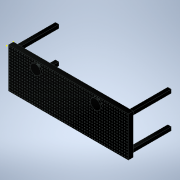
# Autodesk Inventor part: Table_Holed
Saved by Autodesk Inventor 2020 (Build 240168000, 168)
## iProperties
Created: 2019-11-01
Part Number: Table_Holed
Material: Generic
Document SubType Name: Modeling
Designer: Nikol
Density: 1 g/cm^3
Appearance: Gunmetal - Polished
Author: Nikol
Autodesk Inventor part; units mm, degrees
ref_plane "YZ Plane" through (0, 0, 0) normal (1, 0, 0) x (0, 1, 0)
ref_plane "XZ Plane" through (0, 0, 0) normal (0, 1, 0) x (-1, 0, 0)
ref_plane "XY Plane" through (0, 0, 0) normal (0, 0, 1) x (1, 0, 0)
sketch "Sketch1" plane through (0, 0, 0) normal (0, 0, 1) x (1, 0, 0)
  line L0 (0, 0) -> (2400, 0)
  line L1 (2400, 0) -> (2400, -800)
  line L2 (2400, -800) -> (0, -800)
  line L3 (0, -800) -> (0, 0)
  line L4 (0, 0) -> (575, 0)
  line L5 (575, 0) -> (575, -125)
  line L6 (0, 0) -> (1775, 0)
  line L7 (1775, 0) -> (1775, -125)
  circle A0 centre (575, -125) radius 100
  circle A1 centre (1775, -125) radius 100
  dimension "d0" = 2400
  dimension "d1" = 800
  dimension "d2" = 575
  dimension "d3" = 125
  dimension "d4" = 1775
  dimension "d5" = 200
  constraints: 16 end point, 3 perpendicular, 2 centre point, 2 coincident, 2 parallel, 2 point on line, 1 horizontal
  measures "d0" distance of L1.end L2.end
  measures "d1" distance of L0.end L1.end
  measures "d2" distance of L0.start L4.end
  measures "d3" distance of L4.end L5.end
  measures "d4" distance of L0.start L6.end
  measures "d5" diameter of A0
extrude "Extrusion1" add sketch "Sketch1" along normal blind 35 contours A1 | A0
extrude "Extrusion2" add sketch "Sketch1" against normal blind 100
sketch "Sketch2" plane through (575, -125, 35) normal (0, 0, 1) x (1, 0, 0)
  point P0 (-575, 125)
extrude "Extrusion3" add sketch "Sketch1" against normal blind 100 contours A0
extrude "Extrusion4" add sketch "Sketch1" against normal blind 100 contours A1
sketch "Sketch3" plane through (0, 0, -100) normal (0, 0, -1) x (-1, 0, 0)
  point P0 (0, 0)
sketch "Sketch4" plane through (0, 0, -100) normal (0, 0, -1) x (-1, 0, 0)
  line L0 (0, 0) -> (-2400, 0) projected
  line L1 (0, 0) -> (0, -40)
  line L2 (0, -800) -> (0, 0) projected
  line L3 (0, -40) -> (-40, -40)
  line L4 (-40, -40) -> (-110, -40)
  line L5 (-110, -40) -> (-110, -110)
  line L6 (-110, -110) -> (-40, -110)
  line L7 (-40, -110) -> (-40, -40)
  line L8 (-2400, -800) -> (0, -800) projected
  line L9 (0, -800) -> (-40, -800)
  line L10 (0, -760) -> (0, -800)
  line L11 (-40, -760) -> (-110, -760)
  line L12 (-110, -760) -> (-110, -690)
  line L13 (-110, -690) -> (-40, -690)
  line L14 (-40, -690) -> (-40, -760)
  line L15 (-2400, 0) -> (-2400, -800) projected
  line L16 (-2400, 0) -> (-2400, -40)
  line L17 (-2400, -40) -> (-2360, -40)
  line L18 (-2400, -800) -> (-2400, -760)
  line L19 (-2400, -760) -> (-2360, -760)
  line L20 (-2360, -40) -> (-2290, -40)
  line L21 (-2290, -40) -> (-2290, -110)
  line L22 (-2290, -110) -> (-2360, -110)
  line L23 (-2360, -110) -> (-2360, -40)
  line L24 (-2360, -760) -> (-2290, -760)
  line L25 (-2290, -760) -> (-2290, -690)
  line L26 (-2290, -690) -> (-2360, -690)
  line L27 (-2360, -690) -> (-2360, -760)
  dimension "d14" = 40
  dimension "d15" = 40
  dimension "d16" = 70
  dimension "d17" = 70
  dimension "d18" = 40
  dimension "d19" = 40
  dimension "d20" = 70
  dimension "d21" = 70
  dimension "d22" = 40
  dimension "d23" = 40
  dimension "d24" = 70
  dimension "d25" = 70
  dimension "d26" = 70
  dimension "d27" = 70
  constraints: 48 end point, 8 parallel, 6 horizontal, 6 perpendicular, 3 point on line
  measures "d14" distance of L0.start L1.end
  measures "d15" distance of L1.end L3.end
  measures "d16" distance of L6.end L5.end
  measures "d17" distance of L5.end L4.end
  measures "d18" distance of L11.start L10.start
  measures "d19" distance of L9.end L11.start
  measures "d20" distance of L12.end L13.end
  measures "d21" distance of L11.end L12.end
  measures "d22" distance of L0.end L16.end
  measures "d23" distance of L16.end L17.end
  measures "d24" distance of L21.end L22.end
  measures "d25" distance of L20.end L21.end
  measures "d26" distance of L26.end L25.end
  measures "d27" distance of L25.end L24.end
extrude "Extrusion5" add sketch "Sketch4" along normal blind 800 contours L20 L21 L22 L23 | L27 L26 L25 L24 | L7 L6 L5 L4 | L11 L12 L13 L14
sketch "Sketch5" plane through (0, 0, 0) normal (0, 0, 1) x (1, 0, 0)
  circle A0 centre (25, -25) radius 10
  circle A1 centre (25, -75) radius 10
  circle A2 centre (25, -175) radius 10
  circle A3 centre (25, -125) radius 10
  circle A4 centre (25, -375) radius 10
  circle A5 centre (25, -325) radius 10
  circle A6 centre (25, -225) radius 10
  circle A7 centre (25, -275) radius 10
  circle A8 centre (25, -775) radius 10
  circle A9 centre (25, -725) radius 10
  circle A10 centre (25, -625) radius 10
  circle A11 centre (25, -675) radius 10
  circle A12 centre (25, -425) radius 10
  circle A13 centre (25, -475) radius 10
  circle A14 centre (25, -575) radius 10
  circle A15 centre (25, -525) radius 10
  line L0 (2400, -800) -> (0, -800) projected
  circle A16 centre (75, -25) radius 10
  circle A17 centre (75, -75) radius 10
  circle A18 centre (75, -175) radius 10
  circle A19 centre (75, -125) radius 10
  circle A20 centre (75, -375) radius 10
  circle A21 centre (75, -325) radius 10
  circle A22 centre (75, -225) radius 10
  circle A23 centre (75, -275) radius 10
  circle A24 centre (75, -525) radius 10
  circle A25 centre (75, -475) radius 10
  circle A26 centre (75, -425) radius 10
  circle A27 centre (75, -775) radius 10
  circle A28 centre (75, -575) radius 10
  circle A29 centre (75, -625) radius 10
  circle A30 centre (75, -675) radius 10
  circle A31 centre (75, -725) radius 10
  circle A32 centre (125, -625) radius 10
  circle A33 centre (125, -725) radius 10
  circle A34 centre (125, -575) radius 10
  circle A35 centre (125, -525) radius 10
  circle A36 centre (125, -475) radius 10
  circle A37 centre (125, -425) radius 10
  circle A38 centre (125, -375) radius 10
  circle A39 centre (125, -325) radius 10
  circle A40 centre (125, -275) radius 10
  circle A41 centre (125, -225) radius 10
  circle A42 centre (125, -125) radius 10
  circle A43 centre (125, -75) radius 10
  circle A44 centre (125, -25) radius 10
  circle A45 centre (125, -175) radius 10
  circle A46 centre (125, -675) radius 10
  circle A47 centre (125, -775) radius 10
  circle A48 centre (275, -25) radius 10
  circle A49 centre (275, -75) radius 10
  circle A50 centre (275, -175) radius 10
  circle A51 centre (275, -125) radius 10
  circle A52 centre (275, -375) radius 10
  circle A53 centre (275, -325) radius 10
  circle A54 centre (275, -225) radius 10
  circle A55 centre (275, -275) radius 10
  circle A56 centre (275, -525) radius 10
  circle A57 centre (275, -475) radius 10
  circle A58 centre (275, -425) radius 10
  circle A59 centre (275, -775) radius 10
  circle A60 centre (275, -575) radius 10
  circle A61 centre (275, -625) radius 10
  circle A62 centre (275, -675) radius 10
  circle A63 centre (275, -725) radius 10
  circle A64 centre (225, -625) radius 10
  circle A65 centre (225, -725) radius 10
  circle A66 centre (225, -575) radius 10
  circle A67 centre (225, -525) radius 10
  circle A68 centre (225, -475) radius 10
  circle A69 centre (225, -425) radius 10
  circle A70 centre (225, -375) radius 10
  circle A71 centre (225, -325) radius 10
  circle A72 centre (225, -275) radius 10
  circle A73 centre (225, -225) radius 10
  circle A74 centre (225, -125) radius 10
  circle A75 centre (225, -75) radius 10
  circle A76 centre (225, -25) radius 10
  circle A77 centre (225, -175) radius 10
  circle A78 centre (225, -675) radius 10
  circle A79 centre (225, -775) radius 10
  circle A80 centre (175, -325) radius 10
  circle A81 centre (175, -375) radius 10
  circle A82 centre (175, -425) radius 10
  circle A83 centre (175, -575) radius 10
  circle A84 centre (175, -625) radius 10
  circle A85 centre (175, -725) radius 10
  circle A86 centre (175, -775) radius 10
  circle A87 centre (175, -525) radius 10
  circle A88 centre (175, -475) radius 10
  circle A89 centre (175, -675) radius 10
  circle A90 centre (175, -275) radius 10
  circle A91 centre (175, -225) radius 10
  circle A92 centre (175, -125) radius 10
  circle A93 centre (175, -75) radius 10
  circle A94 centre (175, -25) radius 10
  circle A95 centre (175, -175) radius 10
  circle A96 centre (575, -25) radius 10
  circle A97 centre (575, -75) radius 10
  circle A98 centre (575, -175) radius 10
  circle A99 centre (575, -125) radius 10
  circle A100 centre (575, -375) radius 10
  circle A101 centre (575, -325) radius 10
  circle A102 centre (575, -225) radius 10
  circle A103 centre (575, -275) radius 10
  circle A104 centre (575, -525) radius 10
  circle A105 centre (575, -475) radius 10
  circle A106 centre (575, -425) radius 10
  circle A107 centre (575, -775) radius 10
  circle A108 centre (575, -575) radius 10
  circle A109 centre (575, -625) radius 10
  circle A110 centre (575, -675) radius 10
  circle A111 centre (575, -725) radius 10
  circle A112 centre (525, -625) radius 10
  circle A113 centre (525, -725) radius 10
  circle A114 centre (525, -575) radius 10
  circle A115 centre (525, -525) radius 10
  circle A116 centre (525, -475) radius 10
  circle A117 centre (525, -425) radius 10
  circle A118 centre (525, -375) radius 10
  circle A119 centre (525, -325) radius 10
  circle A120 centre (525, -275) radius 10
  circle A121 centre (525, -225) radius 10
  circle A122 centre (525, -125) radius 10
  circle A123 centre (525, -75) radius 10
  circle A124 centre (525, -25) radius 10
  circle A125 centre (525, -175) radius 10
  circle A126 centre (525, -675) radius 10
  circle A127 centre (525, -775) radius 10
  circle A128 centre (475, -325) radius 10
  circle A129 centre (475, -375) radius 10
  circle A130 centre (475, -425) radius 10
  circle A131 centre (475, -575) radius 10
  circle A132 centre (475, -625) radius 10
  circle A133 centre (475, -725) radius 10
  circle A134 centre (475, -775) radius 10
  circle A135 centre (475, -525) radius 10
  circle A136 centre (475, -475) radius 10
  circle A137 centre (475, -675) radius 10
  circle A138 centre (475, -275) radius 10
  circle A139 centre (475, -225) radius 10
  circle A140 centre (475, -125) radius 10
  circle A141 centre (475, -75) radius 10
  circle A142 centre (475, -25) radius 10
  circle A143 centre (475, -175) radius 10
  circle A144 centre (325, -25) radius 10
  circle A145 centre (325, -75) radius 10
  circle A146 centre (375, -475) radius 10
  circle A147 centre (325, -475) radius 10
  circle A148 centre (425, -475) radius 10
  circle A149 centre (325, -425) radius 10
  circle A150 centre (325, -325) radius 10
  circle A151 centre (325, -275) radius 10
  circle A152 centre (325, -225) radius 10
  circle A153 centre (325, -175) radius 10
  circle A154 centre (325, -125) radius 10
  circle A155 centre (325, -375) radius 10
  circle A156 centre (325, -675) radius 10
  circle A157 centre (375, -675) radius 10
  circle A158 centre (325, -725) radius 10
  circle A159 centre (375, -725) radius 10
  circle A160 centre (325, -775) radius 10
  circle A161 centre (375, -775) radius 10
  circle A162 centre (325, -525) radius 10
  circle A163 centre (375, -525) radius 10
  circle A164 centre (325, -575) radius 10
  circle A165 centre (325, -625) radius 10
  circle A166 centre (375, -625) radius 10
  circle A167 centre (375, -575) radius 10
  circle A168 centre (375, -175) radius 10
  circle A169 centre (425, -175) radius 10
  circle A170 centre (425, -125) radius 10
  circle A171 centre (375, -75) radius 10
  circle A172 centre (425, -75) radius 10
  circle A173 centre (375, -25) radius 10
  circle A174 centre (425, -25) radius 10
  circle A175 centre (375, -125) radius 10
  circle A176 centre (375, -425) radius 10
  circle A177 centre (425, -425) radius 10
  circle A178 centre (375, -375) radius 10
  circle A179 centre (425, -375) radius 10
  circle A180 centre (375, -325) radius 10
  circle A181 centre (425, -325) radius 10
  circle A182 centre (375, -275) radius 10
  circle A183 centre (375, -225) radius 10
  circle A184 centre (425, -225) radius 10
  circle A185 centre (425, -275) radius 10
  circle A186 centre (425, -525) radius 10
  circle A187 centre (425, -575) radius 10
  circle A188 centre (425, -625) radius 10
  circle A189 centre (425, -725) radius 10
  circle A190 centre (425, -775) radius 10
  circle A191 centre (425, -675) radius 10
  circle A192 centre (1175, -25) radius 10
  circle A193 centre (1175, -75) radius 10
  circle A194 centre (1175, -175) radius 10
  circle A195 centre (1175, -125) radius 10
  circle A196 centre (1175, -375) radius 10
  circle A197 centre (1175, -325) radius 10
  circle A198 centre (1175, -225) radius 10
  circle A199 centre (1175, -275) radius 10
  circle A200 centre (1175, -525) radius 10
  circle A201 centre (1175, -475) radius 10
  circle A202 centre (1175, -425) radius 10
  circle A203 centre (1175, -775) radius 10
  circle A204 centre (1175, -575) radius 10
  circle A205 centre (1175, -625) radius 10
  circle A206 centre (1175, -675) radius 10
  circle A207 centre (1175, -725) radius 10
  circle A208 centre (1125, -625) radius 10
  circle A209 centre (1125, -725) radius 10
  circle A210 centre (1125, -575) radius 10
  circle A211 centre (1125, -525) radius 10
  circle A212 centre (1125, -475) radius 10
  circle A213 centre (1125, -425) radius 10
  circle A214 centre (1125, -375) radius 10
  circle A215 centre (1125, -325) radius 10
  circle A216 centre (1125, -275) radius 10
  circle A217 centre (1125, -225) radius 10
  circle A218 centre (1125, -125) radius 10
  circle A219 centre (1125, -75) radius 10
  circle A220 centre (1125, -25) radius 10
  circle A221 centre (1125, -175) radius 10
  circle A222 centre (1125, -675) radius 10
  circle A223 centre (1125, -775) radius 10
  circle A224 centre (1075, -325) radius 10
  circle A225 centre (1075, -375) radius 10
  circle A226 centre (1075, -425) radius 10
  circle A227 centre (1075, -575) radius 10
  circle A228 centre (1075, -625) radius 10
  circle A229 centre (1075, -725) radius 10
  circle A230 centre (1075, -775) radius 10
  circle A231 centre (1075, -525) radius 10
  circle A232 centre (1075, -475) radius 10
  circle A233 centre (1075, -675) radius 10
  circle A234 centre (1075, -275) radius 10
  circle A235 centre (1075, -225) radius 10
  circle A236 centre (1075, -125) radius 10
  circle A237 centre (1075, -75) radius 10
  circle A238 centre (1075, -25) radius 10
  circle A239 centre (1075, -175) radius 10
  circle A240 centre (925, -25) radius 10
  circle A241 centre (925, -75) radius 10
  circle A242 centre (975, -475) radius 10
  circle A243 centre (925, -475) radius 10
  circle A244 centre (1025, -475) radius 10
  circle A245 centre (925, -425) radius 10
  circle A246 centre (925, -325) radius 10
  circle A247 centre (925, -275) radius 10
  circle A248 centre (925, -225) radius 10
  circle A249 centre (925, -175) radius 10
  circle A250 centre (925, -125) radius 10
  circle A251 centre (925, -375) radius 10
  circle A252 centre (925, -675) radius 10
  circle A253 centre (975, -675) radius 10
  circle A254 centre (925, -725) radius 10
  circle A255 centre (975, -725) radius 10
  circle A256 centre (925, -775) radius 10
  circle A257 centre (975, -775) radius 10
  circle A258 centre (925, -525) radius 10
  circle A259 centre (975, -525) radius 10
  circle A260 centre (925, -575) radius 10
  circle A261 centre (925, -625) radius 10
  circle A262 centre (975, -625) radius 10
  circle A263 centre (975, -575) radius 10
  circle A264 centre (975, -175) radius 10
  circle A265 centre (1025, -175) radius 10
  circle A266 centre (1025, -125) radius 10
  circle A267 centre (975, -75) radius 10
  circle A268 centre (1025, -75) radius 10
  circle A269 centre (975, -25) radius 10
  circle A270 centre (1025, -25) radius 10
  circle A271 centre (975, -125) radius 10
  circle A272 centre (975, -425) radius 10
  circle A273 centre (1025, -425) radius 10
  circle A274 centre (975, -375) radius 10
  circle A275 centre (1025, -375) radius 10
  circle A276 centre (975, -325) radius 10
  circle A277 centre (1025, -325) radius 10
  circle A278 centre (975, -275) radius 10
  circle A279 centre (975, -225) radius 10
  circle A280 centre (1025, -225) radius 10
  circle A281 centre (1025, -275) radius 10
  circle A282 centre (1025, -525) radius 10
  circle A283 centre (1025, -575) radius 10
  circle A284 centre (1025, -625) radius 10
  circle A285 centre (1025, -725) radius 10
  circle A286 centre (1025, -775) radius 10
  circle A287 centre (1025, -675) radius 10
  circle A288 centre (625, -775) radius 10
  circle A289 centre (625, -675) radius 10
  circle A290 centre (625, -725) radius 10
  circle A291 centre (775, -675) radius 10
  circle A292 centre (775, -775) radius 10
  circle A293 centre (825, -675) radius 10
  circle A294 centre (825, -725) radius 10
  circle A295 centre (875, -675) radius 10
  circle A296 centre (825, -775) radius 10
  circle A297 centre (875, -725) radius 10
  circle A298 centre (875, -775) radius 10
  circle A299 centre (775, -725) radius 10
  circle A300 centre (625, -525) radius 10
  circle A301 centre (625, -475) radius 10
  circle A302 centre (625, -425) radius 10
  circle A303 centre (625, -575) radius 10
  circle A304 centre (675, -575) radius 10
  circle A305 centre (675, -525) radius 10
  circle A306 centre (675, -475) radius 10
  circle A307 centre (725, -425) radius 10
  circle A308 centre (775, -425) radius 10
  circle A309 centre (725, -475) radius 10
  circle A310 centre (775, -475) radius 10
  circle A311 centre (725, -525) radius 10
  circle A312 centre (825, -475) radius 10
  circle A313 centre (775, -525) radius 10
  circle A314 centre (825, -525) radius 10
  circle A315 centre (825, -425) radius 10
  circle A316 centre (625, -625) radius 10
  circle A317 centre (725, -725) radius 10
  circle A318 centre (725, -775) radius 10
  circle A319 centre (725, -675) radius 10
  circle A320 centre (675, -775) radius 10
  circle A321 centre (675, -725) radius 10
  circle A322 centre (675, -675) radius 10
  circle A323 centre (675, -625) radius 10
  circle A324 centre (725, -575) radius 10
  circle A325 centre (725, -625) radius 10
  circle A326 centre (875, -625) radius 10
  circle A327 centre (825, -625) radius 10
  circle A328 centre (775, -625) radius 10
  circle A329 centre (825, -575) radius 10
  circle A330 centre (875, -575) radius 10
  circle A331 centre (875, -525) radius 10
  circle A332 centre (775, -575) radius 10
  circle A333 centre (675, -425) radius 10
  circle A334 centre (775, -375) radius 10
  circle A335 centre (825, -375) radius 10
  circle A336 centre (825, -325) radius 10
  circle A337 centre (775, -325) radius 10
  circle A338 centre (675, -375) radius 10
  circle A339 centre (725, -325) radius 10
  circle A340 centre (725, -375) radius 10
  circle A341 centre (875, -25) radius 10
  circle A342 centre (875, -75) radius 10
  circle A343 centre (875, -475) radius 10
  circle A344 centre (875, -425) radius 10
  circle A345 centre (875, -375) radius 10
  circle A346 centre (875, -325) radius 10
  circle A347 centre (875, -275) radius 10
  circle A348 centre (875, -225) radius 10
  circle A349 centre (875, -175) radius 10
  circle A350 centre (875, -125) radius 10
  circle A351 centre (625, -25) radius 10
  circle A352 centre (625, -75) radius 10
  circle A353 centre (625, -175) radius 10
  circle A354 centre (625, -125) radius 10
  circle A355 centre (675, -225) radius 10
  circle A356 centre (675, -125) radius 10
  circle A357 centre (675, -175) radius 10
  circle A358 centre (725, -125) radius 10
  circle A359 centre (725, -175) radius 10
  circle A360 centre (825, -175) radius 10
  circle A361 centre (775, -125) radius 10
  circle A362 centre (775, -175) radius 10
  circle A363 centre (625, -375) radius 10
  circle A364 centre (625, -325) radius 10
  circle A365 centre (625, -225) radius 10
  circle A366 centre (625, -275) radius 10
  circle A367 centre (675, -325) radius 10
  circle A368 centre (675, -275) radius 10
  circle A369 centre (725, -275) radius 10
  circle A370 centre (725, -225) radius 10
  circle A371 centre (775, -275) radius 10
  circle A372 centre (825, -275) radius 10
  circle A373 centre (775, -225) radius 10
  circle A374 centre (825, -225) radius 10
  circle A375 centre (675, -75) radius 10
  circle A376 centre (675, -25) radius 10
  circle A377 centre (725, -75) radius 10
  circle A378 centre (725, -25) radius 10
  circle A379 centre (825, -125) radius 10
  circle A380 centre (825, -75) radius 10
  circle A381 centre (825, -25) radius 10
  circle A382 centre (775, -25) radius 10
  circle A383 centre (775, -75) radius 10
  circle A384 centre (2375, -25) radius 10
  circle A385 centre (2375, -75) radius 10
  circle A386 centre (2375, -175) radius 10
  circle A387 centre (2375, -125) radius 10
  circle A388 centre (2375, -375) radius 10
  circle A389 centre (2375, -325) radius 10
  circle A390 centre (2375, -225) radius 10
  circle A391 centre (2375, -275) radius 10
  circle A392 centre (2375, -525) radius 10
  circle A393 centre (2375, -475) radius 10
  circle A394 centre (2375, -425) radius 10
  circle A395 centre (2375, -775) radius 10
  circle A396 centre (2375, -575) radius 10
  circle A397 centre (2375, -625) radius 10
  circle A398 centre (2375, -675) radius 10
  circle A399 centre (2375, -725) radius 10
  circle A400 centre (2325, -625) radius 10
  circle A401 centre (2325, -725) radius 10
  circle A402 centre (2325, -575) radius 10
  circle A403 centre (2325, -525) radius 10
  circle A404 centre (2325, -475) radius 10
  circle A405 centre (2325, -425) radius 10
  circle A406 centre (2325, -375) radius 10
  circle A407 centre (2325, -325) radius 10
  circle A408 centre (2325, -275) radius 10
  circle A409 centre (2325, -225) radius 10
  circle A410 centre (2325, -125) radius 10
  circle A411 centre (2325, -75) radius 10
  circle A412 centre (2325, -25) radius 10
  circle A413 centre (2325, -175) radius 10
  circle A414 centre (2325, -675) radius 10
  circle A415 centre (2325, -775) radius 10
  circle A416 centre (2275, -325) radius 10
  circle A417 centre (2275, -375) radius 10
  circle A418 centre (2275, -425) radius 10
  circle A419 centre (2275, -575) radius 10
  circle A420 centre (2275, -625) radius 10
  circle A421 centre (2275, -725) radius 10
  circle A422 centre (2275, -775) radius 10
  circle A423 centre (2275, -525) radius 10
  circle A424 centre (2275, -475) radius 10
  circle A425 centre (2275, -675) radius 10
  circle A426 centre (2275, -275) radius 10
  circle A427 centre (2275, -225) radius 10
  circle A428 centre (2275, -125) radius 10
  circle A429 centre (2275, -75) radius 10
  circle A430 centre (2275, -25) radius 10
  circle A431 centre (2275, -175) radius 10
  circle A432 centre (2125, -25) radius 10
  circle A433 centre (2125, -75) radius 10
  circle A434 centre (2175, -475) radius 10
  circle A435 centre (2125, -475) radius 10
  circle A436 centre (2225, -475) radius 10
  circle A437 centre (2125, -425) radius 10
  circle A438 centre (2125, -325) radius 10
  circle A439 centre (2125, -275) radius 10
  circle A440 centre (2125, -225) radius 10
  circle A441 centre (2125, -175) radius 10
  circle A442 centre (2125, -125) radius 10
  circle A443 centre (2125, -375) radius 10
  circle A444 centre (2125, -675) radius 10
  circle A445 centre (2175, -675) radius 10
  circle A446 centre (2125, -725) radius 10
  circle A447 centre (2175, -725) radius 10
  circle A448 centre (2125, -775) radius 10
  circle A449 centre (2175, -775) radius 10
  circle A450 centre (2125, -525) radius 10
  circle A451 centre (2175, -525) radius 10
  circle A452 centre (2125, -575) radius 10
  circle A453 centre (2125, -625) radius 10
  circle A454 centre (2175, -625) radius 10
  circle A455 centre (2175, -575) radius 10
  circle A456 centre (2175, -175) radius 10
  circle A457 centre (2225, -175) radius 10
  circle A458 centre (2225, -125) radius 10
  circle A459 centre (2175, -75) radius 10
  circle A460 centre (2225, -75) radius 10
  circle A461 centre (2175, -25) radius 10
  circle A462 centre (2225, -25) radius 10
  circle A463 centre (2175, -125) radius 10
  circle A464 centre (2175, -425) radius 10
  circle A465 centre (2225, -425) radius 10
  circle A466 centre (2175, -375) radius 10
  circle A467 centre (2225, -375) radius 10
  circle A468 centre (2175, -325) radius 10
  circle A469 centre (2225, -325) radius 10
  circle A470 centre (2175, -275) radius 10
  circle A471 centre (2175, -225) radius 10
  circle A472 centre (2225, -225) radius 10
  circle A473 centre (2225, -275) radius 10
  circle A474 centre (2225, -525) radius 10
  circle A475 centre (2225, -575) radius 10
  circle A476 centre (2225, -625) radius 10
  circle A477 centre (2225, -725) radius 10
  circle A478 centre (2225, -775) radius 10
  circle A479 centre (2225, -675) radius 10
  circle A480 centre (1825, -775) radius 10
  circle A481 centre (1825, -675) radius 10
  circle A482 centre (1825, -725) radius 10
  circle A483 centre (1975, -675) radius 10
  circle A484 centre (1975, -775) radius 10
  circle A485 centre (2025, -675) radius 10
  circle A486 centre (2025, -725) radius 10
  circle A487 centre (2075, -675) radius 10
  circle A488 centre (2025, -775) radius 10
  circle A489 centre (2075, -725) radius 10
  circle A490 centre (2075, -775) radius 10
  circle A491 centre (1975, -725) radius 10
  circle A492 centre (1825, -525) radius 10
  circle A493 centre (1825, -475) radius 10
  circle A494 centre (1825, -425) radius 10
  circle A495 centre (1825, -575) radius 10
  circle A496 centre (1875, -575) radius 10
  circle A497 centre (1875, -525) radius 10
  circle A498 centre (1875, -475) radius 10
  circle A499 centre (1925, -425) radius 10
  circle A500 centre (1975, -425) radius 10
  circle A501 centre (1925, -475) radius 10
  circle A502 centre (1975, -475) radius 10
  circle A503 centre (1925, -525) radius 10
  circle A504 centre (2025, -475) radius 10
  circle A505 centre (1975, -525) radius 10
  circle A506 centre (2025, -525) radius 10
  circle A507 centre (2025, -425) radius 10
  circle A508 centre (1825, -625) radius 10
  circle A509 centre (1925, -725) radius 10
  circle A510 centre (1925, -775) radius 10
  circle A511 centre (1925, -675) radius 10
  circle A512 centre (1875, -775) radius 10
  circle A513 centre (1875, -725) radius 10
  circle A514 centre (1875, -675) radius 10
  circle A515 centre (1875, -625) radius 10
  circle A516 centre (1925, -575) radius 10
  circle A517 centre (1925, -625) radius 10
  circle A518 centre (2075, -625) radius 10
  circle A519 centre (2025, -625) radius 10
  circle A520 centre (1975, -625) radius 10
  circle A521 centre (2025, -575) radius 10
  circle A522 centre (2075, -575) radius 10
  circle A523 centre (2075, -525) radius 10
  circle A524 centre (1975, -575) radius 10
  circle A525 centre (1875, -425) radius 10
  circle A526 centre (1975, -375) radius 10
  circle A527 centre (2025, -375) radius 10
  circle A528 centre (2025, -325) radius 10
  circle A529 centre (1975, -325) radius 10
  circle A530 centre (1875, -375) radius 10
  circle A531 centre (1925, -325) radius 10
  circle A532 centre (1925, -375) radius 10
  circle A533 centre (2075, -25) radius 10
  circle A534 centre (2075, -75) radius 10
  circle A535 centre (2075, -475) radius 10
  circle A536 centre (2075, -425) radius 10
  circle A537 centre (2075, -375) radius 10
  circle A538 centre (2075, -325) radius 10
  circle A539 centre (2075, -275) radius 10
  circle A540 centre (2075, -225) radius 10
  circle A541 centre (2075, -175) radius 10
  circle A542 centre (2075, -125) radius 10
  circle A543 centre (1825, -25) radius 10
  circle A544 centre (1825, -75) radius 10
  circle A545 centre (1825, -175) radius 10
  circle A546 centre (1825, -125) radius 10
  circle A547 centre (1875, -225) radius 10
  circle A548 centre (1875, -125) radius 10
  circle A549 centre (1875, -175) radius 10
  circle A550 centre (1925, -125) radius 10
  circle A551 centre (1925, -175) radius 10
  circle A552 centre (2025, -175) radius 10
  circle A553 centre (1975, -125) radius 10
  circle A554 centre (1975, -175) radius 10
  circle A555 centre (1825, -375) radius 10
  circle A556 centre (1825, -325) radius 10
  circle A557 centre (1825, -225) radius 10
  circle A558 centre (1825, -275) radius 10
  circle A559 centre (1875, -325) radius 10
  circle A560 centre (1875, -275) radius 10
  circle A561 centre (1925, -275) radius 10
  circle A562 centre (1925, -225) radius 10
  circle A563 centre (1975, -275) radius 10
  circle A564 centre (2025, -275) radius 10
  circle A565 centre (1975, -225) radius 10
  circle A566 centre (2025, -225) radius 10
  circle A567 centre (1875, -75) radius 10
  circle A568 centre (1875, -25) radius 10
  circle A569 centre (1925, -75) radius 10
  circle A570 centre (1925, -25) radius 10
  circle A571 centre (2025, -125) radius 10
  circle A572 centre (2025, -75) radius 10
  circle A573 centre (2025, -25) radius 10
  circle A574 centre (1975, -25) radius 10
  circle A575 centre (1975, -75) radius 10
  circle A576 centre (1275, -175) radius 10
  circle A577 centre (1325, -175) radius 10
  circle A578 centre (1275, -225) radius 10
  circle A579 centre (1325, -225) radius 10
  circle A580 centre (1375, -175) radius 10
  circle A581 centre (1275, -275) radius 10
  circle A582 centre (1275, -325) radius 10
  circle A583 centre (1375, -225) radius 10
  circle A584 centre (1425, -175) radius 10
  circle A585 centre (1425, -225) radius 10
  circle A586 centre (1475, -175) radius 10
  circle A587 centre (1475, -225) radius 10
  circle A588 centre (1325, -275) radius 10
  circle A589 centre (1225, -775) radius 10
  circle A590 centre (1275, -725) radius 10
  circle A591 centre (1275, -675) radius 10
  circle A592 centre (1325, -725) radius 10
  circle A593 centre (1325, -675) radius 10
  circle A594 centre (1275, -775) radius 10
  circle A595 centre (1325, -775) radius 10
  circle A596 centre (1375, -725) radius 10
  circle A597 centre (1375, -675) radius 10
  circle A598 centre (1425, -675) radius 10
  circle A599 centre (1425, -725) radius 10
  circle A600 centre (1475, -675) radius 10
  circle A601 centre (1425, -775) radius 10
  circle A602 centre (1475, -725) radius 10
  circle A603 centre (1475, -775) radius 10
  circle A604 centre (1375, -775) radius 10
  circle A605 centre (1225, -575) radius 10
  circle A606 centre (1225, -725) radius 10
  circle A607 centre (1225, -675) radius 10
  circle A608 centre (1225, -625) radius 10
  circle A609 centre (1425, -475) radius 10
  circle A610 centre (1375, -475) radius 10
  circle A611 centre (1325, -475) radius 10
  circle A612 centre (1475, -475) radius 10
  circle A613 centre (1225, -375) radius 10
  circle A614 centre (1225, -325) radius 10
  circle A615 centre (1225, -275) radius 10
  circle A616 centre (1225, -525) radius 10
  circle A617 centre (1225, -475) radius 10
  circle A618 centre (1225, -425) radius 10
  circle A619 centre (1275, -525) radius 10
  circle A620 centre (1275, -475) radius 10
  circle A621 centre (1325, -325) radius 10
  circle A622 centre (1325, -375) radius 10
  circle A623 centre (1275, -375) radius 10
  circle A624 centre (1275, -425) radius 10
  circle A625 centre (1325, -425) radius 10
  circle A626 centre (1225, -25) radius 10
  circle A627 centre (1225, -225) radius 10
  circle A628 centre (1225, -175) radius 10
  circle A629 centre (1225, -125) radius 10
  circle A630 centre (1225, -75) radius 10
  circle A631 centre (1375, -525) radius 10
  circle A632 centre (1325, -525) radius 10
  circle A633 centre (1275, -575) radius 10
  circle A634 centre (1275, -625) radius 10
  circle A635 centre (1325, -575) radius 10
  circle A636 centre (1425, -525) radius 10
  circle A637 centre (1375, -575) radius 10
  circle A638 centre (1475, -525) radius 10
  circle A639 centre (1325, -625) radius 10
  circle A640 centre (1425, -575) radius 10
  circle A641 centre (1375, -625) radius 10
  circle A642 centre (1475, -575) radius 10
  circle A643 centre (1425, -625) radius 10
  circle A644 centre (1475, -625) radius 10
  circle A645 centre (1275, -125) radius 10
  circle A646 centre (1275, -75) radius 10
  circle A647 centre (1275, -25) radius 10
  circle A648 centre (1325, -125) radius 10
  circle A649 centre (1325, -75) radius 10
  circle A650 centre (1475, -125) radius 10
  circle A651 centre (1375, -125) radius 10
  circle A652 centre (1475, -75) radius 10
  circle A653 centre (1425, -75) radius 10
  circle A654 centre (1475, -25) radius 10
  circle A655 centre (1375, -75) radius 10
  circle A656 centre (1425, -25) radius 10
  circle A657 centre (1375, -25) radius 10
  circle A658 centre (1325, -25) radius 10
  circle A659 centre (1425, -125) radius 10
  circle A660 centre (1375, -375) radius 10
  circle A661 centre (1375, -425) radius 10
  circle A662 centre (1375, -325) radius 10
  circle A663 centre (1425, -375) radius 10
  circle A664 centre (1425, -425) radius 10
  circle A665 centre (1475, -425) radius 10
  circle A666 centre (1375, -275) radius 10
  circle A667 centre (1425, -325) radius 10
  circle A668 centre (1475, -375) radius 10
  circle A669 centre (1425, -275) radius 10
  circle A670 centre (1475, -325) radius 10
  circle A671 centre (1475, -275) radius 10
  circle A672 centre (1775, -525) radius 10
  circle A673 centre (1775, -475) radius 10
  circle A674 centre (1775, -425) radius 10
  circle A675 centre (1775, -575) radius 10
  circle A676 centre (1725, -575) radius 10
  circle A677 centre (1725, -525) radius 10
  circle A678 centre (1775, -375) radius 10
  circle A679 centre (1725, -375) radius 10
  circle A680 centre (1675, -375) radius 10
  circle A681 centre (1725, -425) radius 10
  circle A682 centre (1725, -475) radius 10
  circle A683 centre (1675, -475) radius 10
  circle A684 centre (1675, -525) radius 10
  circle A685 centre (1775, -625) radius 10
  circle A686 centre (1675, -425) radius 10
  circle A687 centre (1625, -425) radius 10
  circle A688 centre (1625, -475) radius 10
  circle A689 centre (1575, -425) radius 10
  circle A690 centre (1525, -425) radius 10
  circle A691 centre (1525, -475) radius 10
  circle A692 centre (1625, -525) radius 10
  circle A693 centre (1575, -525) radius 10
  circle A694 centre (1525, -525) radius 10
  circle A695 centre (1525, -575) radius 10
  circle A696 centre (1575, -575) radius 10
  circle A697 centre (1575, -475) radius 10
  circle A698 centre (1625, -675) radius 10
  circle A699 centre (1625, -775) radius 10
  circle A700 centre (1575, -675) radius 10
  circle A701 centre (1575, -725) radius 10
  circle A702 centre (1525, -675) radius 10
  circle A703 centre (1575, -775) radius 10
  circle A704 centre (1525, -725) radius 10
  circle A705 centre (1525, -775) radius 10
  circle A706 centre (1625, -725) radius 10
  circle A707 centre (1675, -725) radius 10
  circle A708 centre (1675, -775) radius 10
  circle A709 centre (1725, -625) radius 10
  circle A710 centre (1725, -675) radius 10
  circle A711 centre (1725, -725) radius 10
  circle A712 centre (1725, -775) radius 10
  circle A713 centre (1675, -675) radius 10
  circle A714 centre (1525, -625) radius 10
  circle A715 centre (1575, -625) radius 10
  circle A716 centre (1625, -625) radius 10
  circle A717 centre (1625, -575) radius 10
  circle A718 centre (1675, -625) radius 10
  circle A719 centre (1675, -575) radius 10
  circle A720 centre (1525, -225) radius 10
  circle A721 centre (1525, -375) radius 10
  circle A722 centre (1525, -325) radius 10
  circle A723 centre (1525, -275) radius 10
  circle A724 centre (1575, -275) radius 10
  circle A725 centre (1575, -325) radius 10
  circle A726 centre (1575, -375) radius 10
  circle A727 centre (1625, -375) radius 10
  circle A728 centre (1625, -325) radius 10
  circle A729 centre (1675, -325) radius 10
  circle A730 centre (1625, -275) radius 10
  circle A731 centre (1575, -225) radius 10
  circle A732 centre (1575, -175) radius 10
  circle A733 centre (1675, -275) radius 10
  circle A734 centre (1625, -225) radius 10
  circle A735 centre (1725, -325) radius 10
  circle A736 centre (1725, -275) radius 10
  circle A737 centre (1625, -175) radius 10
  circle A738 centre (1675, -225) radius 10
  circle A739 centre (1725, -225) radius 10
  circle A740 centre (1675, -175) radius 10
  circle A741 centre (1725, -175) radius 10
  circle A742 centre (1525, -25) radius 10
  circle A743 centre (1525, -75) radius 10
  circle A744 centre (1525, -175) radius 10
  circle A745 centre (1525, -125) radius 10
  circle A746 centre (1725, -125) radius 10
  circle A747 centre (1675, -125) radius 10
  circle A748 centre (1625, -125) radius 10
  circle A749 centre (1575, -125) radius 10
  circle A750 centre (1725, -75) radius 10
  circle A751 centre (1675, -75) radius 10
  circle A752 centre (1575, -75) radius 10
  circle A753 centre (1625, -75) radius 10
  circle A754 centre (1725, -25) radius 10
  circle A755 centre (1675, -25) radius 10
  circle A756 centre (1625, -25) radius 10
  circle A757 centre (1575, -25) radius 10
  circle A758 centre (1775, -775) radius 10
  circle A759 centre (1775, -675) radius 10
  circle A760 centre (1775, -725) radius 10
  circle A761 centre (1775, -325) radius 10
  circle A762 centre (1775, -275) radius 10
  circle A763 centre (1775, -225) radius 10
  circle A764 centre (1775, -175) radius 10
  circle A765 centre (1775, -125) radius 10
  circle A766 centre (1775, -75) radius 10
  circle A767 centre (1775, -25) radius 10
  point P0 (0, 0)
  point P1 (2400, 0)
  constraints: 768 centre point
extrude "Extrusion6" cut sketch "Sketch5" against normal up to surface (100 mm away)
sketch "Sketch6" plane through (0, 0, -100) normal (0, 0, -1) x (-1, 0, 0)
  line L0 (0, -800) -> (0, 0) projected
  line L1 (0, -800) -> (-2400, -800)
  line L2 (-2400, -800) -> (-2400, 0)
  line L3 (-2400, 0) -> (0, 0)
  line L4 (0, 0) -> (0, -800)
  line L5 (-2360, -110) -> (-2360, -40) projected
  line L6 (-40, -760) -> (-110, -760) projected
  line L7 (-2360, -40) -> (-40, -40)
  line L8 (-40, -40) -> (-40, -760)
  line L9 (-40, -760) -> (-2360, -760)
  line L10 (-2360, -760) -> (-2360, -40)
  constraints: 16 end point, 4 parallel, 2 horizontal, 2 perpendicular
extrude "Extrusion7" cut sketch "Sketch6" against normal blind 70 contours L5 L7 L8 L6 L9 L10
sketch "Sketch7" plane through (0, 0, -30) normal (0, 0, -1) x (-1, 0, 0)
  line L0 (-2360, -40) -> (-40, -40) projected
  line L1 (-110, -110) -> (-110, -40) projected
  line L2 (-40, -40) -> (-110, -40)
  line L3 (-110, -40) -> (-110, -110)
  line L4 (-110, -110) -> (-40, -110)
  line L5 (-40, -110) -> (-40, -40)
  line L6 (-110, -760) -> (-110, -690) projected
  line L7 (-40, -760) -> (-2360, -760) projected
  line L8 (-110, -690) -> (-40, -690)
  line L9 (-40, -690) -> (-40, -760)
  line L10 (-40, -760) -> (-110, -760)
  line L11 (-110, -760) -> (-110, -690)
  line L12 (-2360, -690) -> (-2290, -690) projected
  line L13 (-2360, -760) -> (-2290, -760)
  line L14 (-2290, -760) -> (-2290, -690)
  line L15 (-2290, -690) -> (-2360, -690)
  line L16 (-2360, -690) -> (-2360, -760)
  line L17 (-2290, -110) -> (-2360, -110) projected
  line L18 (-2360, -40) -> (-2290, -40)
  line L19 (-2290, -40) -> (-2290, -110)
  line L20 (-2290, -110) -> (-2360, -110)
  line L21 (-2360, -110) -> (-2360, -40)
  point P0 (0, 0)
  constraints: 32 end point, 8 parallel, 4 horizontal, 4 perpendicular, 2 point on line
extrude "Extrusion8" add sketch "Sketch7" along normal blind 70
body "Solid1"
